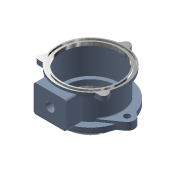
# Autodesk Inventor part: Cylinder_Body
Saved by Autodesk Inventor 2022 Beta2 (Build 260130000, 130) ContinuousBuild 0
## iProperties
Created: 2012-01-26
Part Number: Cylinder_Body
Document SubType Name: Modeling
Designer: mflayler
Manufacturer: Standard
Standards Organization: Custom
Density: 1 g/cm^3
Mass: 132.338 g
Surface Area: 688.081 cm^2
Volume: 132.338 cm^3
Material: Generic
Appearance: Light Steel Blue
Subject: Autodesk Inventor
Author: mflayler
Autodesk Inventor part; units mm, degrees
sketch "Sketch1" plane through (0, 0, 0) normal (0, 0, 1) x (1, 0, 0)
  circle A0 centre (0, 0) radius 55.5
  circle A1 centre (0, 0) radius 47.5
  dimension "d0" = 111
  dimension "d1" = 95
  constraints: 2 centre point, 1 coincident
  measures "d0" diameter of A0
  measures "d1" diameter of A1
extrude "Extrusion1" add sketch "Sketch1" along normal blind 6 draft 3
sketch "Sketch2" plane through (0, 0, 0) normal (0, 0, -1) x (-1, 0, 0)
  circle A0 centre (0, 0) radius 47.5 projected
  circle A1 centre (0, 0) radius 55.5 projected
  circle A2 centre (0, 0) radius 48.5
  dimension "d4" = 97
  constraints: 1 centre point, 1 coincident
  measures "d4" diameter of A2
extrude "Extrusion2" add sketch "Sketch2" along normal blind 41 contours A2
sketch "Sketch3" plane through (0, 0, -41) normal (0, 0, -1) x (-1, 0, 0)
  circle A0 centre (0, 0) radius 48.5 projected
  circle A1 centre (0, 0) radius 40.5
  circle A2 centre (0, 0) radius 60
  dimension "d7" = 120
  dimension "d8" = 81
  constraints: 2 centre point, 2 coincident
  measures "d7" diameter of A2
  measures "d8" diameter of A1
extrude "Extrusion3" add sketch "Sketch3" along normal blind 8.5 contours A0 | A2
sketch "Sketch4" plane through (0, 0, -49.5) normal (0, 0, -1) x (-1, 0, 0)
  circle A0 centre (0, 0) radius 40.5 projected
  circle A1 centre (0, 0) radius 60 projected
  circle A2 centre (0, 0) radius 43
  dimension "d11" = 86
  constraints: 1 centre point, 1 coincident
  measures "d11" diameter of A2
extrude "Extrusion4" add sketch "Sketch4" along normal blind 15 contours A2
ref_plane "Work Plane1" through (0, 0, -2) normal (0, 0, 1) x (1, 0, 0)
sketch "Sketch5" plane through (0, 0, -2) normal (0, 0, 1) x (1, 0, 0)
  line L0 (0, 0) -> (50.5049, -29.159) construction
  line L1 (0, -78.1402) -> (0, 78.1402) projected
  arc A0 (50.5049, -35.659) -> (56.134, -25.909) centre (50.5049, -29.159) ccw
  circle A1 centre (0, 0) radius 48.5 projected
  line L2 (56.134, -25.909) -> (47.3185, -10.64)
  line L3 (50.5049, -35.659) -> (32.8738, -35.659)
  dimension "d15" = 13
  dimension "d16" = 30
  dimension "d17" = 60
  dimension "d18" = 58.318
  constraints: 6 end point, 4 point on circle, 2 coincident, 2 tangent, 1 centre point, 1 other
  measures "d15" diameter of A0
  measures "d16" angle of L3 L0
  measures "d17" angle of L1 L0
  measures "d18" distance of L0.start L0.end
extrude "Extrusion5" add sketch "Sketch5" along normal up to surface (8 mm away) contours A1 L2 A0 L3
fillet "Fillet1" radius 4.5 1 edges at (42.0022, -24.25, -2)
pattern_circular "Circular Pattern1" count 3 over 360 about axis through (0, 0, 0) along (0, 0, -1) of "Extrusion5", "Fillet1"
sketch "Sketch6" plane through (0, 0, 0) normal (1, 0, 0) x (0, 1, 0)
  line L0 (43, -64.5) -> (-43, -64.5) projected
  line L1 (60, -49.5) -> (-60, -49.5) projected
  line L2 (60, -41) -> (-60, -41) projected
  line L3 (-19.3561, 6) -> (55.0151, 6) projected
  line L4 (47.5, 0) -> (47.1856, 6) projected
  line L5 (49.6856, 6) -> (53.6856, 6)
  line L6 (53.6856, 6) -> (53.6856, 3)
  line L7 (53.6856, 3) -> (49.6856, 3)
  line L8 (49.6856, 3) -> (49.6856, 6)
  line L9 (43, -49.5) -> (43, -64.5) projected
  line L10 (43, -63) -> (42, -64.5)
  line L11 (51.1, -49.5) -> (45.2, -49.5)
  line L12 (45.2, -49.5) -> (45.2, -44.8)
  line L13 (45.2, -44.8) -> (51.1, -44.8)
  line L14 (51.1, -44.8) -> (51.1, -49.5)
  line L15 (40.5, -41) -> (40.5, -64.5) projected
  line L16 (40.5, -52.1) -> (41, -43.3)
  line L17 (41, -43.3) -> (47.5, -43.3)
  line L18 (47.5, -43.3) -> (47.5, -41)
  line L19 (0, -78.6) -> (0, 20.1) projected
  dimension "d25" = 4
  dimension "d27" = 3
  dimension "d28" = 1.5
  dimension "d29" = 1
  dimension "d30" = 4.7
  dimension "d31" = 5.9
  dimension "d32" = 4.7
  dimension "d34" = 12.4
  dimension "d35" = 49.3
  dimension "d37" = 0.5
  dimension "d38" = 2.5
  constraints: 24 end point, 5 point on line, 4 parallel, 3 perpendicular, 2 horizontal, 1 vertical, 3 other
  measures "d25" distance of L5.start L5.end
  measures "d27" distance of L5.end L6.end
  measures "d28" distance from line of L0 L10.start
  measures "d29" distance from line of L9 L10.end
  measures "d30" distance of L13.end L11.start
  measures "d31" distance of L11.start L11.end
  measures "d32" distance between parallel lines of L15 L12
  measures "d34" distance from line of L0 L16.start
  measures "d35" distance between parallel lines of L3 L17
  measures "d37" horizontal distance of L16.end L16.start
  measures "d38" distance from line of L4.end L8
revolve "Revolution1" cut sketch "Sketch6" angle 360 about axis through (0, 0, 0) along (0, 0, 1) contours L0 L10 L9 | L15 L1 L16 | L1 L15 L2 L18 L17 L16 | L1 L12 L13 L14 | L3 L6 L7 L8
sketch "Sketch7" plane through (0, 0, -49.5) normal (0, 0, -1) x (-1, 0, 0)
  circle A0 centre (0, 0) radius 51.1 projected
  line L0 (0, 0) -> (-60, 0) construction
  arc A1 (-66.8829, 9.8298) -> (-66.8829, -9.8298) centre (-60, 0) ccw
  circle A2 centre (0, 0) radius 49.6856 projected
  line L1 (-66.8829, -9.8298) -> (-38.1469, -29.951)
  line L2 (-66.8829, 9.8298) -> (-38.1469, 29.951)
  circle A3 centre (0, 0) radius 48.5 projected
  point P0 (-41.1456, -27.8513)
  point P1 (-41.1456, 27.8513)
  dimension "d39" = 60
  dimension "d40" = 35
  dimension "d41" = 12
  constraints: 6 end point, 6 point on circle, 2 point on line, 2 tangent, 1 centre point, 1 coincident, 1 horizontal, 1 other
  measures "d39" distance of L0.start L0.end
  measures "d40" angle of L1 L0
  measures "d41" radius of A1
extrude "Extrusion6" add sketch "Sketch7" against normal blind 12.5 contours L2 A2 L1 A0 | A0 L1 A1 L2 | L2 A3 L1 A2 picked at (-43.7015, 24.2696) picked at (-48.7491, 0)
sketch "Sketch8" plane through (0, 0, -49.5) normal (0, 0, -1) x (-1, 0, 0)
  arc A0 (-44.1318, -25.7603) -> (-44.1318, 25.7603) centre (0, 0) ccw projected
  arc A1 (-38.1469, 29.951) -> (-38.1469, -29.951) centre (0, 0) ccw projected
  circle A2 centre (0, 0) radius 51.1
  line L0 (-38.1469, -29.951) -> (-44.1318, -25.7603)
  line L1 (-38.1469, 29.951) -> (-44.1318, 25.7603)
  constraints: 4 end point, 1 centre point, 1 coincident, 1 concentric
extrude "Extrusion7" cut sketch "Sketch8" against normal up to surface (4.7 mm away) contours A2 L1 A1 L0
fillet "Fillet2" radius 2 1 edges at (48.5, 0, -37)
mirror "Mirror1" about plane through (0, 0, 0) normal (1, 0, 0) of "Extrusion6", "Fillet2", "Extrusion7"
ref_plane "Work Plane2" through (0, -40.5, 0) normal (0, 1, 0) x (-1, 0, 0)
ref_plane "Work Plane3" through (0, -66.8, 0) normal (0, 1, 0) x (-1, 0, 0)
sketch "Sketch9" plane through (0, -66.8, 0) normal (0, 1, 0) x (-1, 0, 0)
  line L0 (-23, -43) -> (23, -43)
  line L1 (27, -39) -> (27, -2)
  line L2 (23, 2) -> (-23, 2)
  line L3 (-27, -2) -> (-27, -39)
  arc A0 (-27, -39) -> (-23, -43) centre (-23, -39) ccw
  arc A1 (23, -43) -> (27, -39) centre (23, -39) ccw
  arc A2 (27, -2) -> (23, 2) centre (23, -2) ccw
  arc A3 (-23, 2) -> (-27, -2) centre (-23, -2) ccw
  line L4 (-42.5286, 0) -> (42.5286, 0) projected
  line L5 (57.7683, -41) -> (-57.7683, -41) projected
  line L6 (0, -53.1598) -> (0, 12.1598) projected
  dimension "d49" = 4
  dimension "d50" = 54
  dimension "d51" = 2
  dimension "d52" = 2
  dimension "d53" = 27
  constraints: 8 end point, 8 point on circle, 8 tangent, 4 centre point, 3 equal radius, 2 parallel, 1 horizontal, 1 perpendicular
  measures "d49" radius of A0
  measures "d50" distance between parallel lines of L1 L3
  measures "d51" distance between parallel lines of L5 L0
  measures "d52" distance between parallel lines of L4 L2
  measures "d53" distance between parallel lines of L6 L3
extrude "Extrusion8" add sketch "Sketch9" along normal up to next
sketch "Sketch10" plane through (0, -66.8, 0) normal (0, -1, 0) x (1, 0, 0)
  line L0 (27, -39) -> (27, -2) projected
  line L1 (23, 2) -> (-23, 2) projected
  point P0 (0, -20.5)
  point P1 (0, 2)
  point P2 (27, -20.5)
  constraints: 2 midpoint, 1 horizontal alignment, 1 vertical alignment
ref_plane "Work Plane16" through (45.5751, -16.588, 0) normal (-0.9396926, 0.3420201, 0) x (-0.3420201, -0.9396926, 0)
ref_plane "Work Plane15" through (0, 0, 0) normal (-0.9396926, 0.3420201, 0) x (0, 0, 1)
hole "Hole9" at (0, -66.8, -20.5) direction (0, 1, 0) diameter 15 end up to surface
hole "Hole11" at (60, 0, -37) direction (0, 0, -1) diameter 10 end through all
equation "\"d53\" = 0.5 * d50"
body "Solid1"
